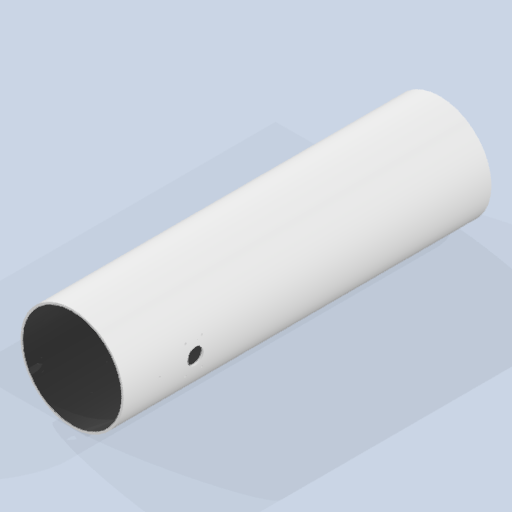
# Autodesk Inventor part: tube
Saved by Autodesk Inventor 2023 (Build 270158000, 158)
## iProperties
Created: 2022-10-12
Part Number: tube
Material: Generic
Document SubType Name: Modeling
Designer: Nathan
Density: 1 g/cm^3
Appearance: Smooth - White
Mass: 7077.61 g
Surface Area: 22432.3 cm^2
Volume: 7077.61 cm^3
Author: Nathan
Autodesk Inventor part; units mm, degrees
ref_plane "YZ Plane" through (0, 0, 0) normal (1, 0, 0) x (0, 1, 0)
ref_plane "XZ Plane" through (0, 0, 0) normal (0, 1, 0) x (-1, 0, 0)
ref_plane "XY Plane" through (0, 0, 0) normal (0, 0, 1) x (1, 0, 0)
sketch "Sketch1" plane through (0, 0, 0) normal (0, 0, 1) x (1, 0, 0)
  circle A0 centre (0, 0) radius 161.1312
  circle A1 centre (0, 0) radius 151.6062
  circle A2 centre (0, 0) radius 153.1937
  circle A3 centre (0, 0) radius 159.5438
  dimension "d2" = 9.525
  dimension "d3" = 303.2125
  dimension "d4" = 322.2625
  dimension "d13" = 306.3875
  dimension "d14" = 319.0875
  dimension "d15" = 6.35
  dimension "d16" = 1.5875
  dimension "d35" = 0
  constraints: 4 centre point, 2 coincident
  measures "d2" radial gap between concentric circles of A1 A0
  measures "d3" diameter of A1
  measures "d4" diameter of A0
  measures "d13" diameter of A2
  measures "d14" diameter of A3
  measures "d15" radial gap between concentric circles of A2 A3
  measures "d16" radial gap between concentric circles of A3 A0
  measures "d35" distance of point (0, 0) A0.centre
extrude "Extrusion1" add sketch "Sketch1" along normal blind 1136.65 contours A3
sketch "Sketch2" plane through (0, 0, 0) normal (1, 0, 0) x (0, 1, 0)
  circle A0 centre (0, 914.4) radius 25.4
  line L0 (159.5438, 1136.65) -> (-159.5438, 1136.65) projected
  circle A1 centre (0, 1025.525) radius 3.175
  circle A2 centre (42.8625, 939.8) radius 3.175
  circle A3 centre (-42.8625, 939.8) radius 3.175
  circle A4 centre (42.8532, 889) radius 3.175
  circle A5 centre (-42.8718, 889) radius 3.175
  point P0 (0, 0)
  point P1 (0, 1136.65)
  dimension "d21" = 50.8
  dimension "d22" = 222.25
  dimension "d23" = 6.35
  dimension "d24" = 111.125
  dimension "d25" = 6.35
  dimension "d26" = 6.35
  dimension "d27" = 85.725
  dimension "d28" = 42.8625
  dimension "d29" = 6.35
  dimension "d30" = 6.35
  dimension "d31" = 85.725
  dimension "d32" = 50.8
  constraints: 6 centre point, 1 midpoint
  measures "d21" diameter of A0
  measures "d22" distance from line of A0.centre L0
  measures "d23" diameter of A1
  measures "d24" distance of point (0, 1136.65) A1.centre
  measures "d25" diameter of A2
  measures "d26" diameter of A3
  measures "d27" distance of A3.centre A2.centre
  measures "d28" horizontal distance of A2.centre point (0, 1136.65)
  measures "d29" diameter of A4
  measures "d30" diameter of A5
  measures "d31" distance of A5.centre A4.centre
  measures "d32" distance of A4.centre A2.centre
extrude "Extrusion3" cut sketch "Sketch2" along normal through all
body "Solid1"
